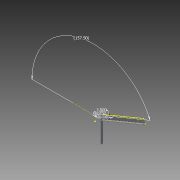
# Autodesk Inventor part: CatapultArmL-Right
Saved by Autodesk Inventor 2013 (Build 170138000, 138)
## iProperties
Created: 2014-01-17
Part Number: CatapultArmL-Right
Material: Generic
Document SubType Name: Modeling
Designer: 215152
Density: 1 g/cm^3
Author: 215152
Autodesk Inventor part; units mm, degrees
ref_plane "YZ Plane" through (0, 0, 0) normal (1, 0, 0) x (0, 1, 0)
ref_plane "XZ Plane" through (0, 0, 0) normal (0, 1, 0) x (-1, 0, 0)
ref_plane "XY Plane" through (0, 0, 0) normal (0, 0, 1) x (1, 0, 0)
ref_plane "Work Plane1" through (0, 0, 0) normal (0, 0, 1) x (1, 0, 0)
sketch "Sketch1" plane through (0, 0, 0) normal (0, 0, 1) x (1, 0, 0)
  line L0 (0, 0) -> (63.5, 0)
  line L1 (63.5, 0) -> (63.5, 482.6)
  line L2 (63.5, 482.6) -> (0, 482.6)
  line L3 (0, 482.6) -> (0, 0)
  line L4 (63.5, 482.6) -> (63.5, 406.4)
  line L5 (63.5, 482.6) -> (139.7, 482.6) construction
  line L6 (63.5, 406.4) -> (-63.5, 406.4)
  line L7 (63.5, 406.4) -> (63.5, 304.8)
  line L8 (63.5, 406.4) -> (165.1, 406.4) construction
  line L9 (63.5, 304.8) -> (1409.7, 304.8)
  line L10 (63.5, 304.8) -> (596.9, 304.8)
  circle A0 centre (596.9, 304.8) radius 88.9
  circle A1 centre (596.9, 304.8) radius 6.35
  line L11 (596.9, 304.8) -> (1174.248, 304.8) construction
  line L12 (596.9, 304.8) -> (538.2336, 280.4996)
  circle A2 centre (538.2336, 280.4996) radius 6.35
  line L13 (596.9, 304.8) -> (614.4999, 312.0901)
  line L14 (596.9, 304.8) -> (615.95, 304.8) construction
  line L15 (614.4999, 312.0901) -> (619.36, 300.3568)
  line L16 (619.36, 300.3568) -> (63.5, 70.1121)
  line L17 (614.4999, 312.0901) -> (609.6398, 323.8234)
  line L18 (614.4999, 312.0901) -> (627.1999, 312.0901) construction
  line L19 (609.6398, 323.8234) -> (63.5, 97.6049)
  line L20 (63.5, 70.1121) -> (63.5, -183.8879)
  line L21 (63.5, 70.1121) -> (317.5, 70.1121) construction
  line L22 (63.5, -183.8879) -> (88.9, -183.8879)
  line L23 (88.9, -183.8879) -> (88.9, 80.6331)
  dimension "d0" = 63.5
  dimension "d1" = 482.6
  dimension "d2" = 76.2
  dimension "d3" = 90
  dimension "d4" = 127
  dimension "d5" = 90
  dimension "d6" = 101.6
  dimension "d7" = 90
  dimension "d8" = 1346.2
  dimension "d9" = 90
  dimension "d10" = 533.4
  dimension "d11" = 177.8
  dimension "d12" = 12.7
  dimension "d14" = 63.5
  dimension "d15" = 12.7
  dimension "d16" = 19.05
  dimension "d17" = 22.5
  dimension "d18" = 12.7
  dimension "d19" = 90
  dimension "d20" = 90
  dimension "d21" = 12.7
  dimension "d22" = 112.5
  dimension "d23" = 591.1375
  dimension "d24" = 90
  dimension "d25" = 254
  dimension "d26" = 90
  dimension "d27" = 25.4
  dimension "d28" = 90
  dimension "d29" = 90
  constraints: 48 end point, 7 horizontal, 7 perpendicular, 5 equal length, 4 point on line, 3 centre point, 3 coincident, 3 collinear, 2 parallel
  measures "d0" distance of L2.end L1.end
  measures "d1" distance of L1.end L0.end
  measures "d2" distance of L1.end L4.end
  measures "d3" angle of L4 L5
  measures "d4" distance of L4.end L6.end
  measures "d5" angle of L4 L6
  measures "d6" distance of L4.end L7.end
  measures "d7" angle of L7 L8
  measures "d8" distance of L7.end L9.end
  measures "d9" angle of L9 L7
  measures "d10" distance of L7.end L10.end
  measures "d11" diameter of A0
  measures "d12" diameter of A1
  measures "d14" distance of L11.start L12.end
  measures "d15" diameter of A2
  measures "d16" distance of L11.start L13.end
  measures "d17" angle of L14 L13
  measures "d18" distance of L13.end L15.end
  measures "d19" angle of L13 L15
  measures "d20" angle of L15 L16
  measures "d21" distance of L13.end L17.end
  measures "d22" angle of L18 L17
  measures "d23" distance of L17.end L19.end
  measures "d24" angle of L19 L17
  measures "d25" distance of L16.end L20.end
  measures "d26" angle of L20 L21
  measures "d27" distance of L20.end L22.end
  measures "d28" angle of L22 L20
  measures "d29" angle of L23 L22
extrude "Extrusion1" add sketch "Sketch1" along normal blind 25.4 contours L1 L16 L23 L22 L20 | L1 L19 A0 L16 | L19 L9 A1 L15 L16 A0 | L19 L17 L13 A1 L9 | L9 A1 L13 L15
sketch "Sketch2" plane through (0, 0, 25.4) normal (0, 0, 1) x (1, 0, 0)
  circle A0 centre (596.9, 304.8) radius 6.35 projected
  line L0 (88.9, 80.6331) -> (619.36, 300.3568) projected
  line L1 (619.36, 300.3568) -> (609.6398, 323.8234) projected
  line L2 (609.6398, 323.8234) -> (63.5, 97.6049) projected
  line L3 (63.5, 97.6049) -> (63.5, -183.8879) projected
  line L4 (63.5, -183.8879) -> (88.9, -183.8879) projected
  line L5 (88.9, -183.8879) -> (88.9, 80.6331) projected
  line L6 (596.9, 304.8) -> (614.4999, 312.0901)
  line L7 (596.9, 304.8) -> (615.95, 304.8) construction
  line L8 (614.4999, 312.0901) -> (604.7797, 335.5567)
  line L9 (614.4999, 312.0901) -> (639.8999, 312.0901) construction
  line L10 (604.7797, 335.5567) -> (624.2201, 288.6236)
  line L11 (624.2201, 288.6236) -> (1203.6463, 288.6236) construction
  line L12 (604.7797, 335.5567) -> (1190.6567, 335.5567) construction
  line L13 (76.2, -183.8879) -> (101.6, -183.8879)
  line L14 (101.6, -183.8879) -> (50.8, -183.8879)
  line L15 (101.6, -183.8879) -> (101.6, 72.1473)
  line L16 (101.6, 72.1473) -> (624.2201, 288.6236)
  line L17 (604.7797, 335.5567) -> (50.8, 106.0907)
  line L18 (604.7797, 335.5567) -> (1204.4031, 335.5567) construction
  line L19 (50.8, 106.0907) -> (50.8, -183.8879)
  point P0 (0, 0)
  dimension "d32" = 22.5
  dimension "d33" = 25.4
  dimension "d34" = 112.5
  dimension "d35" = 50.8
  dimension "d36" = 0
  dimension "d39" = 25.4
  dimension "d40" = 50.8
  dimension "d42" = 157.5
  constraints: 28 end point, 5 horizontal, 3 collinear, 3 equal length, 2 midpoint, 1 parallel, 1 perpendicular
  measures "d32" angle of L7 L6
  measures "d33" distance of L6.end L8.end
  measures "d34" angle of L9 L8
  measures "d35" distance of L8.end L10.end
  measures "d36" distance between parallel lines of L10 L8
  measures "d39" distance of L13.start L13.end
  measures "d40" distance of L13.end L14.end
  measures "d42" angle of L17 L18
extrude "Extrusion2" add sketch "Sketch2" against normal blind 25.4 contours L0 L10 L16 L15 L13 L5 | L2 L3 L14 L19 L17 L8
sketch "Sketch4" plane through (0, 0, 25.4) normal (0, 0, 1) x (1, 0, 0)
  line L0 (604.7797, 335.5567) -> (50.8, 106.0907) projected
  line L1 (50.8, 106.0907) -> (50.8, -183.8879) projected
  line L2 (50.8, -183.8879) -> (101.6, -183.8879) projected
  line L3 (101.6, -183.8879) -> (101.6, 72.1473) projected
  line L4 (76.2, -183.8879) -> (76.2, 116.6118)
  point P0 (0, 0)
  constraints: 2 end point, 1 midpoint, 1 parallel, 1 point on line
extrude "Extrusion3" cut sketch "Sketch4" against normal blind 25.4
sketch "Sketch5" plane through (0, 0, 25.4) normal (0, 0, 1) x (1, 0, 0)
  line L0 (76.2, 116.6118) -> (76.2, -183.8879) projected
  line L1 (76.2, -183.8879) -> (101.6, -183.8879) projected
  line L2 (101.6, -183.8879) -> (101.6, 72.1473) projected
  line L3 (101.6, 72.1473) -> (624.2201, 288.6236) projected
  line L4 (624.2201, 288.6236) -> (604.7797, 335.5567) projected
  line L5 (604.7797, 335.5567) -> (76.2, 116.6118) projected
  circle A0 centre (538.2336, 280.4996) radius 6.35 projected
  circle A1 centre (596.9, 304.8) radius 6.35 projected
  line L6 (101.6, -183.8879) -> (98.425, -183.8879)
  line L7 (101.6, -183.8879) -> (104.775, -183.8879) construction
  line L8 (624.2201, 288.6236) -> (623.005, 291.5569)
  line L9 (624.2201, 288.6236) -> (627.3951, 288.6236) construction
  line L10 (623.005, 291.5569) -> (98.425, 74.2687)
  line L11 (98.425, 74.2687) -> (98.425, -183.8879)
  point P0 (0, 0)
  dimension "d61" = 3.175
  dimension "d62" = 180
  dimension "d63" = 3.175
  dimension "d64" = 112.5
  dimension "d65" = 90
  constraints: 12 end point, 2 equal length, 2 horizontal, 2 perpendicular, 1 collinear
  measures "d61" distance of L1.end L6.end
  measures "d62" angle of L6 L7
  measures "d63" distance of L3.end L8.end
  measures "d64" angle of L9 L8
  measures "d65" angle of L10 L8
extrude "Extrusion4" cut sketch "Sketch5" against normal blind 22.225 contours L5 L4 L10 L11 L1 L0
sketch "Sketch9" plane through (0, 0, 0) normal (0, 0, -1) x (-1, 0, 0)
  line L0 (-76.2, 116.6118) -> (-604.7797, 335.5567) projected
  line L1 (-624.2201, 288.6236) -> (-101.6, 72.1473) projected
  line L2 (19.4758, 63.2352) -> (-215.1896, 160.4367) construction
  line L3 (19.4758, 63.2352) -> (273.4758, 63.2352) construction
  line L4 (-187.2842, 135.1316) -> (-172.0436, 171.9256) construction
  line L5 (-105.5381, 100.1773) -> (-86.2353, 146.7783) construction
  line L6 (-76.2, -183.8879) -> (-76.2, 116.6118) projected
  line L7 (-76.2, 102.8654) -> (-100.2912, 112.8443) construction
  line L8 (-101.6, 72.1473) -> (-76.2, 116.6118) construction
  point P0 (0, 0)
  point P1 (-182.4241, 146.8649)
  dimension "d85" = 254
  dimension "d86" = 157.5
  dimension "d89" = 12.7
  dimension "d91" = 88.9
  dimension "d100" = 19.05
  constraints: 12 end point, 6 point on line, 2 parallel, 1 coincident, 1 equal length, 1 horizontal, 1 perpendicular
  measures "d85" distance of L2.start L2.end
  measures "d86" angle of L3 L2
  measures "d89" distance between parallel lines of L0 L2
  measures "d91" distance between parallel lines of L5 L4
  measures "d100" distance from line of L7.end L8
hole "Hole2" at (182.4241, 146.8649, 0) direction (0, 0, 1) diameter 6.35 end through all
hole "Hole3" at (100.2912, 112.8443, 0) direction (0, 0, 1) diameter 6.35 end through all
body "Solid1"
